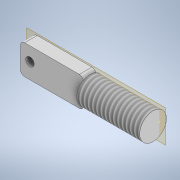
# Autodesk Inventor part: end factor
Saved by Autodesk Inventor 2022 (Build 260153000, 153)
## iProperties
Created: 2021-07-02
Part Number: end factor
Material: Generic
Document SubType Name: Modeling
Designer: 96654
Density: 1 g/cm^3
Appearance: Default
Author: 96654
Autodesk Inventor part; units mm, degrees
ref_plane "YZ Plane" through (0, 0, 0) normal (1, 0, 0) x (0, 1, 0)
ref_plane "XZ Plane" through (0, 0, 0) normal (0, 1, 0) x (-1, 0, 0)
sketch "Sketch1" plane through (0, 0, 0) normal (0, 0, 1) x (1, 0, 0)
  line L0 (-7, -0.2342) -> (-7, 3.2658)
  line L1 (-7, 3.2658) -> (8, 3.2658)
  line L2 (8, 3.2658) -> (8, -3.7342)
  line L3 (8, -3.7342) -> (-7, -3.7342)
  line L4 (-7, -3.7342) -> (-7, -0.2342)
  point P0 (0, 0)
  dimension "d0" = 15
  dimension "d1" = 15
  dimension "d2" = 7
  dimension "d3" = 3.5
  dimension "d4" = 7
  constraints: 10 end point, 3 perpendicular, 1 collinear, 1 point on line, 1 vertical
  measures "d0" distance of L0.end L1.end
  measures "d1" distance of L2.end L3.end
  measures "d2" distance of L1.end L2.end
  measures "d3" distance of L0.start L0.end
  measures "d4" distance from line of point (0, 0) L4
extrude "Extrusion1" add sketch "Sketch1" along normal blind 3
fillet "Fillet1" radius 1 1 edges at (8, 3.2658, 1.5)
fillet "Fillet2" radius 1 1 edges at (8, -3.7342, 1.5)
fillet "Fillet3" radius 1 2 edges at (-7, 3.2658, 1.5) (-7, -3.7342, 1.5)
sketch "Sketch2" plane through (0, 0, 3) normal (0, 0, 1) x (1, 0, 0)
  circle A0 centre (-4.7192, 0) radius 0.9993
  point P0 (0, 0)
  constraints: 1 centre point
extrude "Extrusion2" cut sketch "Sketch2" against normal blind 3
sketch "Sketch3" plane through (8, 2.2658, 3) normal (1, 0, 0) x (0, 0, -1)
  circle A0 centre (1.5431, -2.4625) radius 3.1761
  point P0 (3, -2.2658)
  constraints: 1 centre point
extrude "Extrusion3" add sketch "Sketch3" along normal blind 15
sketch "Sketch4" plane through (23, -0.1967, 1.4569) normal (1, 0, 0) x (0, 0, -1)
  point P0 (1.4569, 0.1967)
sketch "Sketch5" plane through (0, 0, 0) normal (0, 0, 1) x (1, 0, 0)
  point P0 (0, 0)
thread "Thread1" size "M7x1" class "6g" standard "ANSI Metric M Profile" length 15
body "Solid1"
